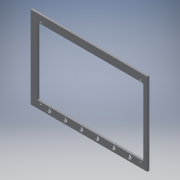
# Autodesk Inventor part: New Bezel
Saved by Autodesk Inventor 2019 (Build 230136000, 136)
## iProperties
Created: 2021-10-07
Part Number: New Bezel
Material: Generic
Document SubType Name: Modeling
Designer: maxwe
Density: 1 g/cm^3
Appearance: Default
Author: maxwe
Autodesk Inventor part; units mm, degrees
ref_plane "YZ Plane" through (0, 0, 0) normal (1, 0, 0) x (0, 1, 0)
ref_plane "Work Plane1" through (-82.5, -59.605, 0) normal (0, 0, 1) x (1, 0, 0)
sketch "Sketch1" plane through (0, 0, 0) normal (0, 0, 1) x (1, 0, 0)
  circle A0 centre (-78.95, -56.05) radius 1.75 projected
  circle A1 centre (78.95, -56.05) radius 1.75 projected
  circle A2 centre (78.95, 56.05) radius 1.75 projected
  circle A3 centre (-78.95, 56.05) radius 1.75 projected
  line L0 (-94.035, 65.475) -> (90.115, 65.475)
  line L1 (90.115, 65.475) -> (90.115, -64.7)
  line L2 (90.115, -64.7) -> (-94.035, -64.7)
  line L3 (-94.035, -64.7) -> (-94.035, 65.475)
  line L4 (-80.31, 46.61) -> (76.39, 46.61) construction
  line L5 (-80.31, -42.49) -> (-80.31, 46.61) construction
  line L6 (76.39, -42.49) -> (-80.31, -42.49) construction
  line L7 (76.39, 46.61) -> (76.39, -42.49) construction
  line L8 (-72.9099, -18.5541) -> (83.1551, -18.5541)
  line L9 (-82.2, -52) -> (82.2, -52) construction
  line L10 (-82.2, -52) -> (82.2, -52) construction
  circle A4 centre (-65.46, -58.76) radius 3.4
  circle A5 centre (-40.06, -58.76) radius 3.4
  circle A6 centre (-14.66, -58.76) radius 3.4
  circle A7 centre (10.74, -58.76) radius 3.4
  circle A8 centre (36.14, -58.76) radius 3.4
  circle A9 centre (61.54, -58.76) radius 3.4
  line L11 (82.5, -51.7) -> (82.5, 51.7) projected
  line L12 (82.2, 52) -> (-82.2, 52) projected
  line L13 (-82.5, 51.7) -> (-82.5, -51.7) projected
  line L14 (-82.2, -52) -> (82.2, -52) projected
  arc A10 (-82.2, 52) -> (-82.5, 51.7) centre (-82.2, 51.7) ccw projected
  arc A11 (82.5, 51.7) -> (82.2, 52) centre (82.2, 51.7) ccw projected
  arc A12 (82.2, -52) -> (82.5, -51.7) centre (82.2, -51.7) ccw projected
  arc A13 (-82.5, -51.7) -> (-82.2, -52) centre (-82.2, -51.7) ccw projected
  line L15 (-82.2, -53.27) -> (82.2, -53.27)
  arc A14 (82.2, -53.27) -> (83.77, -51.7) centre (82.2, -51.7) ccw
  line L16 (83.77, -51.7) -> (83.77, 51.7)
  arc A15 (83.77, 51.7) -> (82.2, 53.27) centre (82.2, 51.7) ccw
  line L17 (82.2, 53.27) -> (-82.2, 53.27)
  arc A16 (-82.2, 53.27) -> (-83.77, 51.7) centre (-82.2, 51.7) ccw
  line L18 (-83.77, 51.7) -> (-83.77, -51.7)
  arc A17 (-83.77, -51.7) -> (-82.2, -53.27) centre (-82.2, -51.7) ccw
  point P0 (-1.96, -64.7)
  dimension "d1" = 130.175
  dimension "d2" = 184.15
  dimension "d3" = 12.7
  dimension "d4" = 6.8
  dimension "d7" = 25.4
  dimension "d18" = 1.27
  constraints: 18 end point, 10 centre point, 8 point on circle, 2 horizontal, 2 parallel, 1 midpoint, 1 perpendicular, 18 other
  measures "d1" distance between parallel lines of L2 L0
  measures "d2" distance between parallel lines of L3 L1
  measures "d3" distance between parallel lines of L2 L9
  measures "d4" diameter of A4
  measures "d7" distance of A4.centre A5.centre
  measures "d18" radial gap between concentric circles of A13 A17
ref_plane "Work Plane2" through (-82.5, -59.605, 0) normal (0, 0, 1) x (1, 0, 0)
extrude "Extrusion2" add sketch "Sketch1" along normal blind 3.175 from surface at 0 contours L0 L1 L2 L3
body "Solid2"
